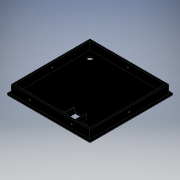
# Autodesk Inventor part: Nanolab CubeDeckel 2
Saved by Autodesk Inventor 2017 (Build 210142000, 142)
## iProperties
Part Number: Nanolab CubeDeckel 2
Material: Generisch
Document SubType Name: Modeling
Designer: David Merges
Density: 1 g/cm^3
Appearance: Eloxiert - schwarz
Author: David Merges
Autodesk Inventor part; units mm, degrees
ref_plane "YZ Plane" through (0, 0, 0) normal (1, 0, 0) x (0, 1, 0)
ref_plane "XZ Plane" through (0, 0, 0) normal (0, 1, 0) x (-1, 0, 0)
ref_plane "XY Plane" through (0, 0, 0) normal (0, 0, 1) x (1, 0, 0)
sketch "Skizze1" plane through (0, 0, 0) normal (0, 0, 1) x (1, 0, 0)
  line L0 (-50.8, 50.8) -> (50.8, 50.8)
  line L1 (50.8, 50.8) -> (50.8, -50.8)
  line L2 (50.8, -50.8) -> (-50.8, -50.8)
  line L3 (-50.8, -50.8) -> (-50.8, 50.8)
  line L4 (50.8, -50.8) -> (-50.8, 50.8) construction
  point P0 (0, 0)
  point P1 (0, 0)
  dimension "d0" = 101.6
  dimension "d1" = 101.6
  constraints: 10 end point, 2 parallel, 1 coincident, 1 horizontal, 1 midpoint, 1 perpendicular
  measures "d0" distance of L1.end L2.end
  measures "d1" distance of L0.end L1.end
extrude "Extrusion1" add sketch "Skizze1" against normal blind 2.0066
fillet "Rundung1" radius 2.0066 4 edges at (50.8, -50.8, -1.0033) (50.8, 50.8, -1.0033) (-50.8, 50.8, -1.0033) (-50.8, -50.8, -1.0033)
fillet "Rundung2" radius 2.0066 8 edges at (-50.2123, -50.2123, -2.0066) (-50.8, 0, -2.0066) (-50.2123, 50.2123, -2.0066) (0, 50.8, -2.0066) (50.2123, 50.2123, -2.0066) (50.8, 0, -2.0066) (50.2123, -50.2123, -2.0066) (0, -50.8, -2.0066)
sketch "Skizze2" plane through (0, 0, 0) normal (0, 0, 1) x (1, 0, 0)
  line L0 (-47.5996, 47.5996) -> (47.5996, 47.5996)
  line L1 (47.5996, 47.5996) -> (47.5996, -47.5996)
  line L2 (47.5996, -47.5996) -> (-47.5996, -47.5996)
  line L3 (-47.5996, -47.5996) -> (-47.5996, 47.5996)
  line L4 (47.5996, -47.5996) -> (-47.5996, 47.5996) construction
  line L5 (-45.593, 45.593) -> (45.593, 45.593)
  line L6 (45.593, 45.593) -> (45.593, -45.593)
  line L7 (45.593, -45.593) -> (-45.593, -45.593)
  line L8 (-45.593, -45.593) -> (-45.593, 45.593)
  line L9 (-45.593, -45.593) -> (45.593, 45.593) construction
  point P0 (0, 0)
  point P1 (0, 0)
  dimension "d6" = 95.1992
  dimension "d7" = 2.0066
  constraints: 20 end point, 4 parallel, 3 perpendicular, 2 horizontal, 2 midpoint, 2 point on line, 1 coincident
  measures "d6" distance of L0.start L0.end
  measures "d7" distance between parallel lines of L1 L6
extrude "Extrusion2" add sketch "Skizze2" along normal blind 9.9822
sketch "Skizze3" plane through (47.5996, -47.5996, 0) normal (1, 0, 0) x (0, 0, -1)
  line L0 (0, 95.1992) -> (0, 0) projected
  line L1 (0, 95.1992) -> (-9.9822, 95.1992) projected
  line L2 (-9.9822, 0) -> (-9.9822, 95.1992) projected
  line L3 (0, 0) -> (-9.9822, 0) projected
  line L4 (0, 47.5996) -> (-4.7752, 47.5996) construction
  line L5 (0, 95.1992) -> (0, 0) construction
  dimension "d10" = 4.7752
  constraints: 2 end point, 1 horizontal, 1 midpoint
  measures "d10" distance of L4.start L4.end
hole "Bohrung1" at (47.5996, 0, 4.7752) direction (-1, 0, 0) diameter 1.941 depth 7.675 tip angle 118 thread size "3-48 UNC" class "2B" standard "ANSI Unified Screw Threads"
pattern_circular "Runde Anordnung1" count 3 over 180 about axis through (0, 0, -10) along (0, 0, 1) of "Bohrung1"
sketch "Skizze4" plane through (-47.5996, -47.5996, 0) normal (0, -1, 0) x (1, 0, 0)
  line L0 (95.1992, 0) -> (0, 0) projected
  line L1 (95.1992, 0) -> (95.1992, 9.9822) projected
  line L2 (0, 9.9822) -> (95.1992, 9.9822) projected
  line L3 (0, 0) -> (0, 9.9822) projected
  line L4 (47.5996, 0) -> (47.5996, 4.7752) construction
  line L5 (22.1996, 4.7752) -> (72.9996, 4.7752) construction
  dimension "d21" = 4.7752
  dimension "d22" = 50.8
  constraints: 4 end point, 1 horizontal, 1 midpoint, 1 vertical
  measures "d21" distance of L4.end L4.start
  measures "d22" distance of L5.start L5.end
hole "Bohrung2" at (-25.4, -47.5996, 4.7752) at (25.4, -47.5996, 4.7752) direction (0, 1, 0) diameter 1.941 depth 7.675 tip angle 118 thread size "3-48 UNC" class "2B" standard "ANSI Unified Screw Threads"
sketch "Skizze5" plane through (0, 0, -2.0066) normal (0, 0, -1) x (-1, 0, 0)
  line L0 (37.5031, -37.5031) -> (-37.5031, -37.5031) construction
  line L1 (-37.5031, -37.5031) -> (-37.5031, 37.5031) construction
  line L2 (-37.5031, 37.5031) -> (37.5031, 37.5031) construction
  line L3 (37.5031, 37.5031) -> (37.5031, -37.5031) construction
  line L4 (-37.5031, 37.5031) -> (37.5031, -37.5031) construction
  point P0 (0, 0)
  point P1 (0, 0)
  dimension "d30" = 75.0062
  constraints: 10 end point, 2 parallel, 2 perpendicular, 1 coincident, 1 horizontal, 1 midpoint
  measures "d30" distance of L0.start L0.end
hole "Bohrung3" at (-37.5031, 37.5031, -2.0066) direction (0, 0, 1) diameter 6 end through all
sketch "Skizze6" plane through (0, 0, 0) normal (0, 0, 1) x (1, 0, 0)
  circle A0 centre (-37.5031, 37.5031) radius 3 projected
  line L0 (-48.7934, 48.7934) -> (-48.7934, -48.7934) projected
  line L1 (48.7934, 48.7934) -> (-48.7934, 48.7934) projected
  line L2 (48.7934, -48.7934) -> (48.7934, 48.7934) projected
  line L3 (-48.7934, -48.7934) -> (48.7934, -48.7934) projected
  circle A1 centre (-37.5031, 37.5031) radius 3.45
  circle A2 centre (-37.5031, 37.5031) radius 1.4986
  point P0 (0, 0)
  dimension "d38" = 2.9972
  dimension "d39" = 6.9
  constraints: 2 centre point, 2 coincident
  measures "d38" diameter of A2
  measures "d39" diameter of A1
extrude "Extrusion3" add sketch "Skizze6" along normal blind 5 contours A0 | A1
pattern_circular "Runde Anordnung2" count 4 over 360 about axis through (0, 0, -10) along (0, 0, 1) of "Bohrung3", "Extrusion3"
sketch "Skizze7" plane through (0, 0, 0) normal (0, 0, 1) x (1, 0, 0)
  circle A0 centre (37.5031, 37.5031) radius 3 projected
  circle A1 centre (37.5031, -37.5031) radius 3 projected
  circle A2 centre (-37.5031, -37.5031) radius 3 projected
  circle A3 centre (-37.5031, 37.5031) radius 3 projected
  line L0 (-48.7934, 48.7934) -> (-48.7934, -48.7934) projected
  line L1 (48.7934, 48.7934) -> (-48.7934, 48.7934) projected
  line L2 (48.7934, -48.7934) -> (48.7934, 48.7934) projected
  line L3 (-48.7934, -48.7934) -> (48.7934, -48.7934) projected
  line L4 (7.9248, -28.2956) -> (24.638, -28.2956)
  line L5 (24.638, -28.2956) -> (24.638, -44.2214)
  line L6 (24.638, -44.2214) -> (7.9248, -44.2214)
  line L7 (7.9248, -44.2214) -> (7.9248, -28.2956)
  line L8 (9.9314, -30.3022) -> (22.6314, -30.3022)
  line L9 (22.6314, -30.3022) -> (22.6314, -43.0022)
  line L10 (22.6314, -43.0022) -> (9.9314, -43.0022)
  line L11 (9.9314, -43.0022) -> (9.9314, -30.3022)
  line L12 (16.2814, -28.2956) -> (16.2814, -30.3022) construction
  circle A4 centre (2.7814, -36.6522) radius 1.4986
  circle A5 centre (2.7814, -36.6522) radius 3.4163
  circle A6 centre (29.7814, -36.6522) radius 1.4986
  circle A7 centre (29.7814, -36.6522) radius 3.4163
  line L13 (9.9314, -43.0022) -> (22.6314, -30.3022) construction
  line L14 (29.7814, -36.6522) -> (2.7814, -36.6522) construction
  line L15 (50.8, -48.7934) -> (48.7934, -48.7934) projected
  arc A8 (48.7934, -50.8) -> (50.8, -48.7934) centre (48.7934, -48.7934) ccw projected
  line L16 (48.7934, -48.7934) -> (48.7934, -50.8) projected
  line L17 (50.8, 48.7934) -> (50.8, -48.7934) projected
  line L18 (48.7934, -50.8) -> (-48.7934, -50.8) projected
  point P0 (0, 0)
  point P1 (16.2814, -36.6522)
  dimension "d46" = 12.7
  dimension "d49" = 1.2192
  dimension "d51" = 6.8326
  dimension "d52" = 27
  dimension "d53" = 2.9972
  dimension "d58" = 2.0066
  dimension "d59" = 2.0066
  dimension "d61" = 14.1478
  dimension "d70" = 28.1686
  dimension "d71" = 21.0186
  dimension "d72" = 27
  constraints: 22 end point, 4 centre point, 4 midpoint, 4 parallel, 4 perpendicular, 3 horizontal, 2 coincident, 2 equal radius
  measures "d46" distance of L8.start L8.end
  measures "d49" distance between parallel lines of L10 L6
  measures "d51" diameter of A7
  measures "d52" distance of L14.start L14.end
  measures "d53" diameter of A4
  measures "d58" distance between parallel lines of L7 L11
  measures "d59" distance between parallel lines of L4 L8
  measures "d61" distance from line of L14 L16.end
  measures "d70" distance between parallel lines of L9 L17
  measures "d71" distance from line of A6.centre L17
  measures "d72" distance of A4.centre A6.centre
extrude "Extrusion4" add sketch "Skizze7" along normal blind 5.0038 contours L4 L5 L6 L7 | A4 | A5 | A6 | A7
sketch "Skizze8" plane through (0, 0, -2.0066) normal (0, 0, -1) x (-1, 0, 0)
  circle A0 centre (-29.7814, -36.6522) radius 2.5019
  circle A1 centre (-2.7814, -36.6522) radius 2.5019
  circle A2 centre (-2.7814, -36.6522) radius 3.4163 projected
  circle A3 centre (-29.7814, -36.6522) radius 3.4163 projected
  point P0 (0, 0)
  dimension "d64" = 5.0038
  constraints: 3 coincident, 2 centre point, 1 equal radius
  measures "d64" diameter of A1
extrude "Extrusion5" cut sketch "Skizze8" against normal blind 2.0066 contours A0 | A1
sketch "Skizze10" plane through (2.7814, -36.6522, 5.0038) normal (0, 0, 1) x (1, 0, 0)
  circle A0 centre (0, 0) radius 3.4163 projected
  circle A1 centre (27, 0) radius 3.4163 projected
  circle A2 centre (0, 0) radius 1.5875
  circle A3 centre (27, 0) radius 3.4163 projected
  circle A4 centre (27, 0) radius 1.5875
  point P0 (-2.7814, 36.6522)
  dimension "d67" = 3.175
  constraints: 2 centre point, 2 coincident, 1 equal radius
  measures "d67" diameter of A2
extrude "Extrusion6" cut sketch "Skizze10" against normal blind 3.4798 contours A2 | A4
sketch "Skizze12" plane through (0, 0, 9.9822) normal (0, 0, 1) x (1, 0, 0)
  line L0 (45.593, -45.593) -> (45.593, 45.593) construction
  line L1 (45.593, 45.593) -> (-45.593, 45.593) construction
  line L2 (-45.593, 45.593) -> (-45.593, -45.593) construction
  line L3 (-45.593, -45.593) -> (45.593, -45.593) construction
  circle A0 centre (-37.5031, 37.5031) radius 3.45 construction
  circle A1 centre (-37.5031, -37.5031) radius 3.45 construction
  circle A2 centre (37.5031, -37.5031) radius 3.45 construction
  circle A3 centre (37.5031, 37.5031) radius 3.45 construction
  circle A4 centre (29.7814, -36.6522) radius 3.4163 construction
  circle A5 centre (2.7814, -36.6522) radius 3.4163 construction
  line L4 (24.638, -28.2956) -> (24.638, -44.2214) construction
  line L5 (24.638, -44.2214) -> (7.9248, -44.2214) construction
  line L6 (7.9248, -44.2214) -> (7.9248, -28.2956) construction
  line L7 (7.9248, -28.2956) -> (24.638, -28.2956) construction
  line L8 (-47.625, 47.625) -> (47.625, 47.625) construction
  line L9 (47.625, 47.625) -> (47.625, -47.625) construction
  line L10 (47.625, -47.625) -> (-47.625, -47.625) construction
  line L11 (-47.625, -47.625) -> (-47.625, 47.625) construction
  line L12 (47.625, -47.625) -> (-47.625, 47.625) construction
  line L13 (45.593, -45.593) -> (-45.593, -45.593) construction
  line L14 (-45.593, 45.593) -> (45.593, 45.593) construction
  line L15 (-45.593, -45.593) -> (45.593, 45.593) construction
  line L16 (9.9314, -27.775) -> (22.6314, -27.775)
  line L17 (22.6314, -27.775) -> (22.6314, -41.375)
  line L18 (22.6314, -41.375) -> (9.9314, -41.375)
  line L19 (9.9314, -41.375) -> (9.9314, -27.775)
  line L20 (22.6314, -30.3022) -> (22.6314, -43.0022) projected
  line L21 (9.9314, -43.0022) -> (9.9314, -30.3022) projected
  circle A6 centre (37.5031, 37.5031) radius 1.4986 projected
  circle A7 centre (37.5031, 37.5031) radius 3.45
  circle A8 centre (37.5031, -37.5031) radius 1.4986 projected
  circle A9 centre (37.5031, -37.5031) radius 3.45
  circle A10 centre (29.7814, -36.6522) radius 1.5875 projected
  circle A11 centre (29.7814, -36.6522) radius 3.4163
  line L22 (7.9248, -28.2956) -> (7.9248, -44.2214) projected
  line L23 (24.638, -28.2956) -> (24.638, -44.2214) projected
  line L24 (7.9248, -44.2214) -> (24.638, -44.2214)
  line L25 (24.638, -44.2214) -> (24.638, -40.875)
  line L26 (24.638, -40.875) -> (7.9248, -40.875)
  line L27 (7.9248, -40.875) -> (7.9248, -44.2214)
  line L28 (7.9248, -28.2956) -> (8.9248, -28.2956)
  line L29 (8.9248, -28.2956) -> (8.9248, -40.875)
  line L30 (8.9248, -40.875) -> (7.9248, -40.875)
  line L31 (7.9248, -40.875) -> (7.9248, -28.2956)
  circle A12 centre (2.7814, -36.6522) radius 1.5875 projected
  circle A13 centre (2.7814, -36.6522) radius 3.4163
  circle A14 centre (-37.5031, -37.5031) radius 3 projected
  circle A15 centre (-37.5031, -37.5031) radius 3.45
  circle A16 centre (-37.5031, 37.5031) radius 1.4986 projected
  circle A17 centre (-37.5031, 37.5031) radius 3.45
  point P0 (0, 0)
  point P1 (0, 0)
  point P2 (16.2814, -41.375)
  dimension "d76" = 95.25
  dimension "d77" = 12.7
  dimension "d78" = 13.6
  dimension "d79" = 6.25
  dimension "d80" = 63.9064
  dimension "d84" = 1
  dimension "d87" = 2.8464
  dimension "d88" = 3.3464
  constraints: 36 end point, 8 parallel, 6 centre point, 6 coincident, 5 concentric, 5 perpendicular, 4 horizontal, 3 midpoint, 2 point on line
  measures "d76" distance of L8.start L8.end
  measures "d77" distance of L16.start L16.end
  measures "d78" distance of L16.end L17.end
  measures "d79" distance between parallel lines of L18 L10
  measures "d80" distance from line of point (16.281, -41.375) L11
  measures "d84" distance between parallel lines of L31 L29
  measures "d87" distance between parallel lines of L18 L5
  measures "d88" distance between parallel lines of L5 L26
extrude "Extrusion7" cut sketch "Skizze12" against normal through all contours L16 L17 L26 L19 | L26 L17 L18 L19
extrude "Extrusion8" cut sketch "Skizze12" against normal up to surface (9.9822 mm away) contours L26 L17 L18 L19 | L19 L18 L17 L26 L23 L24 L22 | L26 L22 L28 L29 | A7 | A9 | A10 | A11 | A12 | A13 | A14 | A15 | A17
equation "\"d59\" = d58"
